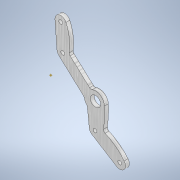
# Autodesk Inventor part: アーノン
Saved by Autodesk Inventor 2022.2 (Build 262287030, 287C)
## iProperties
Created: 2022-01-29
Part Number: アーノン
Material: Aluminum 7075
Document SubType Name: Modeling
Designer: acps
Density: 2.81 g/cm^3
Appearance: Satin - Brushed Heavy
Author: acps
Autodesk Inventor part; units mm, degrees
ref_plane "YZ Plane" through (0, 0, 0) normal (1, 0, 0) x (0, 1, 0)
ref_plane "XZ Plane" through (0, 0, 0) normal (0, 1, 0) x (-1, 0, 0)
ref_plane "XY Plane" through (0, 0, 0) normal (0, 0, 1) x (1, 0, 0)
sketch "Sketch1" plane through (0, 0, 0) normal (0, 0, 1) x (1, 0, 0)
  circle A0 centre (7.8339, 40) radius 4.5
  circle A1 centre (7.8339, 40) radius 1.5
  circle A2 centre (9.4447, 20) radius 4.5
  circle A3 centre (9.4447, 20) radius 1.5
  circle A4 centre (34.6118, -20) radius 4.5
  circle A5 centre (34.6118, -20) radius 1.5
  circle A6 centre (53.9309, -32) radius 4.5
  circle A7 centre (53.9309, -32) radius 1.5
  line L0 (3.3484, 39.6387) -> (4.9593, 19.6387)
  circle A8 centre (35, 0) radius 7.025
  line L1 (6.404, 16.6828) -> (26.106, -1.3771)
  line L2 (28.617, -6.3449) -> (30.1377, -20.4813)
  line L3 (32.2374, -23.8226) -> (51.5565, -35.8226)
  circle A9 centre (35, 0) radius 4.025
  line L4 (14.3908, 21.5707) -> (31.3649, 6.0114)
  arc A10 (14.3908, 21.5707) -> (11.951, 41.8166) centre (-20.0705, 27.6877) ccw
  arc A11 (57.4046, -29.1394) -> (41.0725, -17.3055) centre (26.5269, -54.5671) ccw
  arc A12 (41.0725, -17.3055) -> (42.0194, 0.2811) centre (-51.9053, -3.4806) ccw
  arc A13 (26.106, -1.3771) -> (28.617, -6.3449) centre (35, 0) ccw
  dimension "d9" = 14.05
  dimension "d10" = 8.05
  dimension "d11" = 35
  dimension "d12" = 40
  dimension "d13" = 94
  dimension "d15" = 7
  constraints: 18 point on circle, 14 centre point, 14 tangent, 10 end point, 1 coincident, 1 parallel, 15 other
  measures "d9" diameter of A8
  measures "d10" diameter of A9
  measures "d11" radius of A10
  measures "d12" radius of A11
  measures "d13" radius of A12
  measures "d15" distance of A11.end A4.centre
extrude "Extrusion1" add sketch "Sketch1" against normal blind 3
fillet "Fillet1" radius 2 5 edges at (26.106, -1.3771, -1.5) (28.617, -6.3449, -1.5) (14.3908, 21.5707, -1.5) (41.0725, -17.3055, -1.5) (31.3649, 6.0114, -1.5)
body "Solid1"
